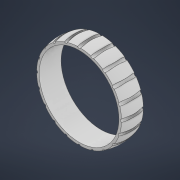
# Autodesk Inventor part: Wheel Outer
Saved by Autodesk Inventor 2022.1 (Build 261234000, 234)
## iProperties
Created: 2021-10-11
Part Number: Wheel Outer
Material: Generic
Document SubType Name: Modeling
Designer: Santiago Martínez
Mass: 8.68 g
Surface Area: 84.8479 cm^2
Volume: 8.68 cm^3
Density: 1 g/cm^3
Appearance: Default
Author: Santiago Martínez
Autodesk Inventor part; units mm, degrees
ref_plane "YZ Plane" through (0, 0, 0) normal (1, 0, 0) x (0, 1, 0)
ref_plane "XZ Plane" through (0, 0, 0) normal (0, 1, 0) x (-1, 0, 0)
ref_plane "XY Plane" through (0, 0, 0) normal (0, 0, 1) x (1, 0, 0)
sketch "Profile S" plane through (0, 0, 0) normal (0, 0, 1) x (1, 0, 0)
  circle A0 centre (0, 0) radius 32 projected
  circle A1 centre (0, 0) radius 31
  circle A2 centre (0, 0) radius 33
  dimension "d0" = 62
  dimension "d1" = 66
  constraints: 2 centre point, 2 coincident
  measures "d0" diameter of A1
  measures "d1" diameter of A2
extrude "Outer Wall" add sketch "Profile S" along normal blind 17 contours A0 | A2
sketch "Sketch3" plane through (0, 0, 17) normal (0, 0, 1) x (1, 0, 0)
  circle A0 centre (0, 0) radius 31 projected
  circle A1 centre (0, 0) radius 33 projected
  circle A2 centre (0, 0) radius 33 projected
  circle A3 centre (0, 0) radius 33 projected
  arc A4 (3.9319, 34.0887) -> (-3.9319, 34.0887) centre (0, 31) ccw
  arc A5 (-6.8291, 32.2857) -> (-3.9319, 34.0887) centre (-7.8638, 37.1774) ccw
  arc A6 (3.9319, 34.0887) -> (6.8291, 32.2857) centre (7.8638, 37.1774) ccw
  point P0 (6.8291, 32.2857)
  dimension "d20" = 31
  dimension "d21" = 10
  dimension "d22" = 5
  constraints: 8 point on circle, 4 tangent, 3 centre point, 2 horizontal alignment, 1 vertical alignment
  measures "d20" distance of point (0, 0) A4.centre
  measures "d21" diameter of A4
  measures "d22" radius of A5
sketch "Sketch4" plane through (0, 0, 0) normal (1, 0, 0) x (0, 1, 0)
  line L0 (33, 17) -> (-33, 17) projected
  line L1 (33, 0) -> (-33, 0) projected
  line L2 (33, 0) -> (-33, 0) projected
  line L3 (33, 17) -> (-33, 17) projected
  arc A0 (33, 0) -> (33, 17) centre (4.2294, 8.5) ccw
  line L4 (33, 17) -> (33, 0)
  line L5 (0, -3.4) -> (0, 20.4) projected
  point P0 (0, 0)
  dimension "d28" = 30
  constraints: 2 end point, 2 point on circle, 1 centre point, 1 perpendicular
  measures "d28" radius of A0
revolve "Revolution1" add sketch "Sketch4" angle 360 about axis through (0, 0, -10) along (0, 0, 1) contours A0 L4
sketch "Sketch5" plane through (0, 0, 17) normal (0, 0, 1) x (1, 0, 0)
  circle A0 centre (0, 0) radius 31 projected
  circle A1 centre (0, 0) radius 33 projected
  circle A2 centre (0, 0) radius 33 projected
  circle A3 centre (0, 33.5) radius 1.25
  point P0 (-1.1369, 32.9804)
  point P1 (1.1369, 32.9804)
  dimension "d30" = 2.5
  dimension "d33" = 33.5
  constraints: 1 centre point, 1 vertical alignment
  measures "d30" diameter of A3
  measures "d33" distance of point (0, 0) A3.centre
extrude "Extrusion5" cut sketch "Sketch5" against normal blind 17 contours A3 A1 | A1 A3 picked at (0, 32.7485) picked at (-0.0397, 33.58)
pattern_circular "Circular Pattern4" count 20 over 360 about axis through (0, 0, 8.5) along (0, 0, -1) of "Extrusion5"
body "Solid1"
